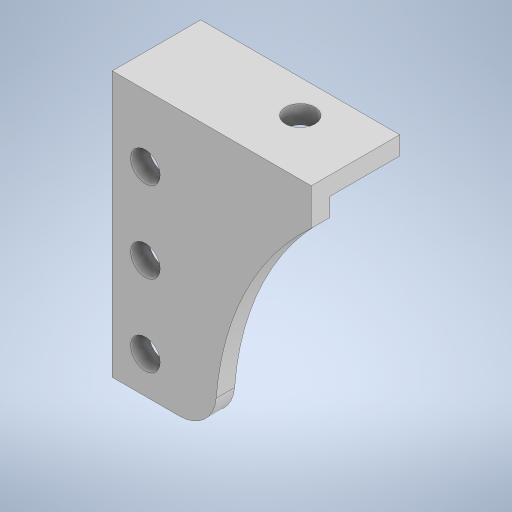
# Autodesk Inventor part: 1-19
Saved by Autodesk Inventor 2024.2 (Build 282272000, 272)
## iProperties
Created: 2024-11-02
Part Number: 1-19
Material: Generic
Document SubType Name: Modeling
Designer: Jimena Brenes
Density: 1 g/cm^3
Appearance: Default
Author: Jimena Brenes
Autodesk Inventor part; units mm, degrees
ref_plane "YZ Plane" through (0, 0, 0) normal (1, 0, 0) x (0, 1, 0)
ref_plane "XZ Plane" through (0, 0, 0) normal (0, 1, 0) x (-1, 0, 0)
ref_plane "XY Plane" through (0, 0, 0) normal (0, 0, 1) x (1, 0, 0)
sketch "Sketch1" plane through (0, 0, 0) normal (0, 0, 1) x (1, 0, 0)
  line L0 (0, 0) -> (0, 5)
  line L1 (0, 5) -> (-27, 5)
  line L2 (-27, 5) -> (-27, -31)
  line L3 (-27, -31) -> (-13, -31)
  arc A0 (0, 0) -> (-12.903, -26.393) centre (26.9732, -29.5372) ccw
  arc A1 (-17.8875, -31) -> (-12.903, -26.393) centre (-17.8875, -26) ccw
  dimension "d3" = 5
  dimension "d4" = 27
  dimension "d5" = 36
  dimension "d6" = 14
  dimension "d9" = 40
  dimension "d10" = 10
  constraints: 8 end point, 4 point on circle, 3 perpendicular, 2 centre point, 2 tangent, 1 point on line, 1 vertical
  measures "d3" distance of L0.start L0.end
  measures "d4" distance of L0.end L1.end
  measures "d5" distance of L1.end L2.end
  measures "d6" distance of L2.end L3.end
  measures "d9" radius of A0
  measures "d10" diameter of A1
extrude "Extrusion1" add sketch "Sketch1" along normal blind 2.5
sketch "Sketch4" plane through (-27, 5, 0) normal (0, 1, 0) x (1, 0, 0)
  circle A0 centre (18, -7.5) radius 2
  line L0 (0, 0) -> (0, -2.5) projected
  line L1 (27, 0) -> (0, 0) projected
  point P0 (0, -12)
  dimension "d20" = 4
  dimension "d21" = 18
  dimension "d22" = 7.5
  constraints: 1 centre point
  measures "d20" diameter of A0
  measures "d21" distance from line of L0 A0.centre
  measures "d22" distance from line of L1 A0.centre
hole "Hole1" at (-9, 5, 7.5) direction (0, -1, 0) diameter 4 end through all
sketch "Sketch5" plane through (0, 0, 2.5) normal (0, 0, 1) x (1, 0, 0)
  line L0 (-22.5, -4) -> (-22.5, -26) construction
  circle A0 centre (-22.5, -4) radius 2
  circle A1 centre (-22.5, -15) radius 2
  circle A2 centre (-22.5, -26) radius 2
  line L1 (-27, 5) -> (0, 5) projected
  line L2 (-27, 5) -> (-27, -31) projected
  point P0 (0, 0)
  point P1 (-27, 2.5)
  dimension "d30" = 4
  dimension "d31" = 4
  dimension "d32" = 4
  dimension "d33" = 11
  dimension "d34" = 9
  dimension "d35" = 11
  dimension "d36" = 4.5
  constraints: 3 centre point, 2 coincident, 2 end point, 1 midpoint, 1 vertical
  measures "d30" diameter of A0
  measures "d31" diameter of A1
  measures "d32" diameter of A2
  measures "d33" distance of L0.start A1.centre
  measures "d34" distance from line of L1 L0.start
  measures "d35" distance of A1.centre L0.end
  measures "d36" distance from line of L2 L0.start
hole "Hole2" at (-22.5, -4, 2.5) at (-22.5, -15, 2.5) at (-22.5, -26, 2.5) direction (0, 0, -1) diameter 4 end through all
sketch "Sketch6" plane through (-27, 5, 0) normal (0, 1, 0) x (1, 0, 0)
  line L0 (27, -2.5) -> (0, -2.5)
  line L1 (0, -2.5) -> (0, 9.5)
  line L2 (0, 9.5) -> (27, 9.5)
  line L3 (27, 9.5) -> (27, -2.5)
  line L4 (27, -2.5) -> (0, -2.5) projected
  line L5 (27, 0) -> (0, 0)
  dimension "d44" = 0
  dimension "d45" = 12
  dimension "d46" = 27
  constraints: 10 end point, 2 parallel, 2 perpendicular, 1 horizontal, 1 point on line
  measures "d44" distance between parallel lines of L4 L0
  measures "d45" distance between parallel lines of L2 L0
  measures "d46" distance between parallel lines of L3 L1
extrude "Extrusion3" add sketch "Sketch6" against normal blind 2.5 contours L5 L1 L2 L3
sketch "Sketch7" plane through (-27, 5, 2.5) normal (0, 1, 0) x (1, 0, 0)
  circle A0 centre (18, 7.5) radius 2
  line L0 (27, 0) -> (0, 0) projected
  line L1 (0, 12) -> (0, 0) projected
  point P0 (27, 2.5)
  dimension "d49" = 4
  dimension "d50" = 7.5
  dimension "d51" = 18
  constraints: 1 centre point
  measures "d49" diameter of A0
  measures "d50" distance from line of L0 A0.centre
  measures "d51" distance from line of L1 A0.centre
hole "Hole3" at (-9, 5, -5) direction (0, -1, 0) diameter 4 end through all
body "Solid1"
